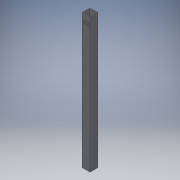
# Autodesk Inventor part: mounting part 2
Saved by Autodesk Inventor 2018 (Build 220112000, 112)
## iProperties
Created: 2019-01-26
Part Number: mounting part 2
Material: Generic
Document SubType Name: Modeling
Designer: s-4008082
Density: 1 g/cm^3
Appearance: Default
Author: s-4008082
Autodesk Inventor part; units mm, degrees
ref_plane "YZ Plane" through (0, 0, 0) normal (1, 0, 0) x (0, 1, 0)
ref_plane "XZ Plane" through (0, 0, 0) normal (0, 1, 0) x (-1, 0, 0)
ref_plane "XY Plane" through (0, 0, 0) normal (0, 0, 1) x (1, 0, 0)
sketch "Sketch1" plane through (0, 0, 0) normal (0, 1, 0) x (-1, 0, 0)
  line L0 (0, 0) -> (25.4, 0)
  line L1 (25.4, 0) -> (25.4, 25.4)
  line L2 (25.4, 25.4) -> (0, 25.4)
  line L3 (0, 25.4) -> (0, 0)
  line L4 (23.749, 23.749) -> (1.651, 23.749)
  line L5 (1.651, 23.749) -> (1.651, 1.651)
  line L6 (1.651, 1.651) -> (23.749, 1.651)
  line L7 (23.749, 1.651) -> (23.749, 23.749)
  dimension "d0" = 25.4
  dimension "d1" = 25.4
  dimension "d2" = 1.651
  dimension "d3" = 1.651
  dimension "d4" = 1.651
  dimension "d5" = 1.651
  constraints: 16 end point, 4 parallel, 2 horizontal, 2 perpendicular
  measures "d0" distance of L1.end L2.end
  measures "d1" distance of L0.end L1.end
  measures "d2" distance between parallel lines of L1 L7
  measures "d3" distance between parallel lines of L0 L6
  measures "d4" distance between parallel lines of L3 L5
  measures "d5" distance between parallel lines of L2 L4
extrude "Extrusion1" add sketch "Sketch1" along normal blind 431.8
sketch "Sketch2" plane through (-25.4, 0, 0) normal (-1, 0, 0) x (0, 0, 1)
  circle A0 centre (12.7, 38.1) radius 2.5797
  circle A1 centre (12.7, 63.5) radius 2.5797
  circle A2 centre (12.7, 88.9) radius 2.5797
  line L0 (0, 0) -> (0, 431.8) projected
  line L1 (0, 0) -> (25.4, 0) projected
  dimension "d8" = 5.1594
  dimension "d9" = 12.7
  dimension "d10" = 12.7
  dimension "d11" = 12.7
  dimension "d12" = 5.1594
  dimension "d13" = 5.1594
  dimension "d14" = 25.4
  dimension "d15" = 50.8
  dimension "d16" = 38.1
  constraints: 3 centre point
  measures "d8" diameter of A0
  measures "d9" distance from line of L0 A0.centre
  measures "d10" distance from line of L0 A1.centre
  measures "d11" distance from line of L0 A2.centre
  measures "d12" diameter of A1
  measures "d13" diameter of A2
  measures "d14" distance of A1.centre A0.centre
  measures "d15" distance of A0.centre A2.centre
  measures "d16" distance from line of L1 A0.centre
extrude "Extrusion2" cut sketch "Sketch2" against normal blind 25.4
sketch "Sketch3" plane through (-25.4, 0, 25.4) normal (0, 0, 1) x (1, 0, 0)
  circle A0 centre (12.7, 381) radius 9.525
  line L0 (0, 431.8) -> (25.4, 431.8) projected
  line L1 (25.4, 0) -> (25.4, 431.8) projected
  dimension "d19" = 19.05
  dimension "d20" = 50.8
  dimension "d26" = 12.7
  constraints: 1 centre point
  measures "d19" diameter of A0
  measures "d20" distance from line of L0 A0.centre
  measures "d26" distance from line of L1 A0.centre
extrude "Extrusion3" cut sketch "Sketch3" against normal blind 25.4
sketch "Sketch5" plane through (-25.4, 0, 25.4) normal (0, 0, 1) x (1, 0, 0)
  circle A0 centre (12.7, 357.1875) radius 2.5797
  circle A1 centre (12.7, 404.8125) radius 2.5797
  circle A2 centre (12.7, 381) radius 9.525 projected
  line L0 (25.4, 0) -> (25.4, 431.8) projected
  dimension "d27" = 23.8125
  dimension "d28" = 23.8125
  dimension "d29" = 5.1594
  dimension "d30" = 5.1594
  dimension "d31" = 12.7
  dimension "d32" = 12.7
  constraints: 2 centre point
  measures "d27" distance of A2.centre A1.centre
  measures "d28" distance of A2.centre A0.centre
  measures "d29" diameter of A0
  measures "d30" diameter of A1
  measures "d31" distance from line of L0 A0.centre
  measures "d32" distance from line of L0 A1.centre
extrude "Extrusion4" cut sketch "Sketch5" against normal blind 76.2 contours A0 | A1
equation "\"d3\" = d2"
equation "\"d4\" = d2"
equation "\"d5\" = d2"
equation "\"d10\" = d9"
equation "\"d11\" = d9"
equation "\"d12\" = d8"
equation "\"d13\" = d8"
equation "\"d28\" = d27"
equation "\"d30\" = d29"
body "Solid1"
